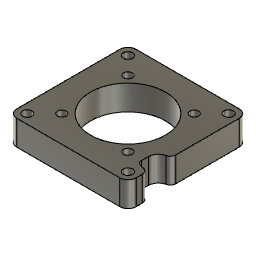
X_Axis_Bracket (Autodesk Fusion 360 design; units mm, degrees)
Autodesk Fusion 360 part; units mm, degrees
sketch "Sketch1" plane through (0, 0, 0) normal (0, 0, 1) x (1, 0, 0)
  line L0 (-27.8831, 24.1702) -> (-27.8831, -24.1098)
  circle A0 centre (23.6169, -23.5198) radius 2.2
  arc A1 (24.2069, -27.9198) -> (28.0169, -24.1098) centre (24.2069, -24.1098) ccw
  line L1 (-24.0731, -27.9198) -> (24.2069, -27.9198)
  circle A2 centre (23.6169, 23.5802) radius 2.2
  line L2 (24.2069, 27.9802) -> (-24.0731, 27.9802)
  spline S0 degree 5 poles (28.0169, -21.3028) (28.0169, -21.1603) (28.0055, -20.8859) (27.9539, -20.5067) (27.8203, -20.0644) (27.5661, -19.6103) (27.2491, -19.2452) (26.8901, -18.9576) (26.4983, -18.7351) (26.0664, -18.5646) (25.5813, -18.4304) (25.0343, -18.3121) (24.4296, -18.1826) (23.7979, -18.0051) (23.1967, -17.7339) (22.6942, -17.3216) (22.4247, -16.8443) (22.3203, -16.389) (22.2971, -16.0405) (22.2971, -15.8549) knots -1 -1 -1 -1 -1 -1 -0.933333 -0.866667 -0.8 -0.733333 -0.666667 -0.6 -0.533333 -0.466667 -0.4 -0.333333 -0.266667 -0.2 -0.133333 -0.066667 0 0 0 0 0 0
  circle A3 centre (-23.4831, 23.5802) radius 2.2
  arc A4 (25.9741, -8.0941) -> (28.0169, -5.6032) centre (25.4769, -5.6032) ccw
  arc A5 (25.9741, -8.0941) -> (22.2971, -12.5777) centre (26.8691, -12.5777) ccw
  circle A6 centre (0.0669, 0.0302) radius 17.5
  arc A7 (-24.0731, 27.9802) -> (-27.8831, 24.1702) centre (-24.0731, 24.1702) ccw
  line L3 (22.2971, -15.8549) -> (22.2971, -12.5777)
  arc A8 (28.0169, 24.1702) -> (24.2069, 27.9802) centre (24.2069, 24.1702) ccw
  line L4 (28.0169, -5.6032) -> (28.0169, 24.1702)
  circle A9 centre (-23.4831, -23.5198) radius 2.2
  arc A10 (-27.8831, -24.1098) -> (-24.0731, -27.9198) centre (-24.0731, -24.1098) ccw
  line L5 (28.0169, -24.1098) -> (28.0169, -21.3028)
  circle A11 centre (-15.4271, 15.5242) radius 2.032
  circle A12 centre (15.5609, 15.5242) radius 2.032
  circle A13 centre (15.5609, -15.4638) radius 2.032
  circle A14 centre (-15.4271, -15.4638) radius 2.032
  circle A15 centre (-15.4271, -15.4638) radius 4.064
  circle A16 centre (15.5609, -15.4638) radius 4.064
  circle A17 centre (15.5609, 15.5242) radius 4.064
  circle A18 centre (-15.4271, 15.5242) radius 4.064
  dimension "d1" = 4.064
  dimension "d2" = 4.064
  dimension "d3" = 4.064
  dimension "d4" = 4.064
  dimension "d7" = 8.128
  dimension "d8" = 8.128
  dimension "d9" = 8.128
  dimension "d10" = 8.128
  constraint concentric A14 A15
  constraint concentric A13 A16
  constraint concentric A12 A17
  constraint concentric A11 A18
  measures "d1" diameter of A11
  measures "d2" diameter of A12
  measures "d3" diameter of A13
  measures "d4" diameter of A14
  measures "d7" diameter of A15
  measures "d8" diameter of A16
  measures "d9" diameter of A17
  measures "d10" diameter of A18
extrude "Extrude1" add sketch "Sketch1" along normal blind 11.684 contours L0 A1 L1 L2 S0 A4 A5 A7 L3 A8 L4 A10 L5 | A15 | A16 | A17 | A18
extrude "Extrude2" cut sketch "Sketch1" along normal blind 3.556 contours A15 | A16 | A17 | A18
